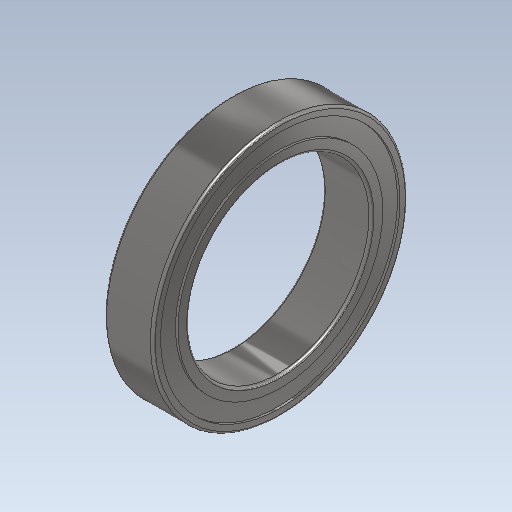
# Autodesk Inventor part: B6702ZZ
Saved by Autodesk Inventor 2020.2 (Build 242310000, 310)
## iProperties
Part Number: B6702ZZ
Material: 鋼、炭素鋼
Catalog Web Link: www.cadenas.de
Description: B6_ _ _ZZ, SB6_ _ _ZZ-Deep Groove Ball Bearings - Double Shield Type
Vendor: MISUMI
Document SubType Name: Modeling
Designer: partserver
Manufacturer: MISUMI
Mass: 5.05558 g
Surface Area: 8.18207 cm^2
Volume: 0.644023 cm^3
Density: 7.85 g/cm^3
Appearance: 半つや出し
Category: PARTsolutions
Company: MISUMI
PSOL_IDENT_0: {$CADENAS_DATA\23d-libs\misumi\metric\12_bearing_holders\sb6010zz.prj},172 {VTYP=3D},{NB=B6702ZZ},{L
PSOL_IDENT_1: INA=B6702ZZ},{NN=B6_ _ _ZZ, SB6_ _ _ZZ},{DATE=22.10.2019 07:39:52},{GEOMDATE=22.10.2019 06:26:04},{V
PSOL_IDENT_2: ERSION=},{LINEID=110},{WBVAR=TS},{WBNUMERIC=}  {NB=B6702ZZ},{LINA=B6702ZZ},{KT=DUMMY},{PN=B6702ZZ},{
PSOL_IDENT_3: TS=},{TS1= '', 'Steel', 'S', 'Stainless Steel'},{MAT=52100 Bearing Steel},{BN=6702ZZ},{DD=15},{D=21}
PSOL_IDENT_4: ,{B=4},{RR=0.2},{CR=0.93},{COR=0.58},{CRS=0.93},{CRSS=0.74},{CORS=0.58},{CORSS=0.46},{DD1=1.00},{R1=
PSOL_IDENT_5: 1.00},{R2=1.0},{DSMIN=15.4},{DSMAX=16.86},{DS1=16.86},{DDHH=19.7},{R=0.2},{MASS=4},{MASS11=4},{AA=3.
PSOL_IDENT_6: 6000},{BB=0.6500},{CC=0.9300},{TYS=w/o Retaining Ring}
NN: B6_ _ _ZZ, SB6_ _ _ZZ
NT: Deep Groove Ball Bearings - Double Shield Type
NB: B6702ZZ
NBSYN: $PN.
LINA: B6702ZZ
PN: B6702ZZ
TS: Steel
MAT: 52100 Bearing Steel
BN: 6702ZZ
DD: 15
D: 21
B: 4
RR: 0.2
CR: 0.93
COR: 0.58
DSMIN: 15.4
DSMAX: 16.86
DDHH: 19.7
R: 0.2
MASS: 4
SUPPLIER: MISUMI
ARTICLENO: B6702ZZ
BOMINFO: B6702ZZ
CREATOR: CADENAS GmbH
d1: 0.000 mm
Title: B6702ZZ
Author: Cadenas PARTsolutions
Comments: Deep Groove Ball Bearings - Double Shield Type
Autodesk Inventor part; units mm, degrees
sketch "Sketch_1" plane through (0, 0, 0) normal (0, 0, 1) x (1, 0, 0)
  line L0 (4, 0) -> (0, 0)
  arc A0 (0, 7.7) -> (0.2, 7.5) centre (0.2, 7.7) ccw
  line L1 (0.2, 7.5) -> (3.8, 7.5)
  arc A1 (3.8, 7.5) -> (4, 7.7) centre (3.8, 7.7) ccw
  line L2 (4, 7.7) -> (4, 8.43)
  line L3 (4, 8.43) -> (3.8, 8.43)
  line L4 (3.8, 8.43) -> (3.8, 9.85)
  line L5 (3.8, 9.85) -> (4, 9.85)
  line L6 (4, 9.85) -> (4, 10.3)
  arc A2 (4, 10.3) -> (3.8, 10.5) centre (3.8, 10.3) ccw
  line L7 (3.8, 10.5) -> (0.2, 10.5)
  arc A3 (0.2, 10.5) -> (0, 10.3) centre (0.2, 10.3) ccw
  line L8 (0, 10.3) -> (0, 9.85)
  line L9 (0, 9.85) -> (0.2, 9.85)
  line L10 (0.2, 9.85) -> (0.2, 8.43)
  line L11 (0.2, 8.43) -> (0, 8.43)
  line L12 (0, 8.43) -> (0, 7.7)
  constraints: 26 end point, 8 point on circle, 4 centre point
revolve "Revolution1" add sketch "Sketch_1" angle 360 about axis through (4, 0, 0) along (1, 0, 0)
ref_plane "center_point_XY" through (2, 0, 0) normal (1, 0, 0) x (0, 0, -1)
ref_plane "center_point_YZ" through (2, 0, 0) normal (0, 0, -1) x (0, 1, 0)
ref_plane "center_point_ZX" through (2, 0, 0) normal (0, 1, 0) x (1, 0, 0)
ref_plane "to_housing_XY" through (0, 0, 0) normal (1, 0, 0) x (0, 0, -1)
ref_plane "to_housing_YZ" through (0, 0, 0) normal (0, 0, -1) x (0, 1, 0)
ref_plane "to_housing_ZX" through (0, 0, 0) normal (0, 1, 0) x (1, 0, 0)
ref_plane "to_ring_XY" through (3.6, 0, 0) normal (1, 0, 0) x (0, 0, -1)
ref_plane "to_ring_YZ" through (3.6, 0, 0) normal (0, 0, -1) x (0, 1, 0)
ref_plane "to_ring_ZX" through (3.6, 0, 0) normal (0, 1, 0) x (1, 0, 0)
body "Solid1"
